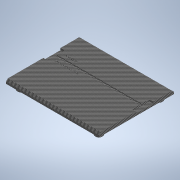
# Autodesk Inventor part: BasePlate2
Saved by Autodesk Inventor 2020 (Build 240168000, 168)
## iProperties
Created: 2026-05-21
Part Number: BasePlate2
Material: Generic
Document SubType Name: Modeling
Designer: sutan
Density: 1 g/cm^3
Appearance: Default
Author: sutan
Autodesk Inventor part; units mm, degrees
ref_plane "YZ Plane" through (0, 0, 0) normal (1, 0, 0) x (0, 1, 0)
ref_plane "XZ Plane" through (0, 0, 0) normal (0, 1, 0) x (-1, 0, 0)
ref_plane "XY Plane" through (0, 0, 0) normal (0, 0, 1) x (1, 0, 0)
sketch "Sketch1" plane through (0, 0, 0) normal (0, 1, 0) x (-1, 0, 0)
  line L0 (22.2515, 145.4131) -> (-225.0785, 145.4131)
  line L1 (-225.0785, 145.4131) -> (-225.0785, 345.4131)
  line L2 (-225.0785, 345.4131) -> (22.2515, 345.4131)
  line L3 (22.2515, 345.4131) -> (22.2515, 145.4131)
  point P0 (0, 0)
  dimension "d0" = 247.33
  dimension "d1" = 200
  constraints: 8 end point, 2 parallel, 1 horizontal, 1 perpendicular
  measures "d0" distance of L1.end L2.end
  measures "d1" distance of L0.end L1.end
extrude "Extrusion1" add sketch "Sketch1" along normal blind 10
sketch "Sketch2" plane through (0, 10, 0) normal (0, 1, 0) x (1, 0, 0)
  line L0 (225.0785, -145.4131) -> (-22.2515, -145.4131) projected
  line L1 (-22.2515, -245.9131) -> (-11.7515, -245.9131)
  line L2 (-11.7515, -245.9131) -> (-11.7515, -200.4131)
  line L3 (-11.7515, -200.4131) -> (-22.2515, -200.4131)
  line L4 (-22.2515, -200.4131) -> (-22.2515, -245.9131)
  line L5 (225.0785, -245.9131) -> (214.5785, -245.9131)
  line L6 (214.5785, -245.9131) -> (214.5785, -200.4131)
  line L7 (214.5785, -200.4131) -> (225.0785, -200.4131)
  line L8 (225.0785, -200.4131) -> (225.0785, -245.9131)
  line L9 (225.0785, -345.4131) -> (225.0785, -145.4131) projected
  line L10 (-22.2515, -145.4131) -> (-22.2515, -345.4131) projected
  point P0 (0, 0)
  point P1 (-9.7325, -245.4131)
  dimension "d4" = 100
  dimension "d5" = 10.5
  dimension "d6" = 45.5
  dimension "d7" = 10.5
  dimension "d8" = 45.5
  dimension "d36" = 0
  dimension "d37" = 0
  dimension "d38" = 0.5
  constraints: 16 end point, 4 parallel, 2 horizontal, 2 perpendicular
  measures "d4" distance from line of L0 point (-9.733, -245.413)
  measures "d5" distance of L3.end L2.end
  measures "d6" distance of L2.end L1.end
  measures "d7" distance of L6.end L7.end
  measures "d8" distance of L5.end L6.end
  measures "d36" distance between parallel lines of L9 L8
  measures "d37" distance between parallel lines of L10 L4
  measures "d38" distance from line of point (-9.733, -245.413) L1
extrude "Extrusion2" cut sketch "Sketch2" against normal blind 5
sketch "Sketch3" plane through (0, 0, 0) normal (0, -1, 0) x (1, 0, 0)
  circle A0 centre (-2.2515, 325.4131) radius 10
  line L0 (-22.2515, 345.4131) -> (225.0785, 345.4131) projected
  line L1 (-22.2515, 145.4131) -> (-22.2515, 345.4131) projected
  line L2 (225.0785, 345.4131) -> (225.0785, 145.4131) projected
  line L3 (225.0785, 145.4131) -> (-22.2515, 145.4131) projected
  circle A1 centre (205.0785, 325.4131) radius 10
  circle A2 centre (205.0785, 165.4131) radius 10
  circle A3 centre (-2.2515, 165.4131) radius 10
  point P0 (0, 0)
  dimension "d11" = 20
  dimension "d12" = 20
  dimension "d13" = 20
  dimension "d16" = 20
  dimension "d17" = 20
  dimension "d18" = 20
  constraints: 4 centre point
  measures "d11" diameter of A0
  measures "d12" distance from line of L0 A0.centre
  measures "d13" distance from line of L1 A0.centre
  measures "d16" diameter of A1
  measures "d17" diameter of A2
  measures "d18" diameter of A3
extrude "Extrusion3" add sketch "Sketch3" along normal blind 15 contours A0 | A1 | A2 | A3
chamfer "Chamfer1" distance 2.5 angle 45 4 edges at (-12.2515, -15, 325.4131) (-12.2515, -15, 165.4131) (195.0785, -15, 325.4131) (195.0785, -15, 165.4131)
sketch "Sketch5" plane through (0, 10, 0) normal (0, 1, 0) x (1, 0, 0)
  line L0 (62.0301, -192.0815) -> (43.5025, -192.0815) construction
  line L1 (43.5025, -192.0815) -> (43.5025, -188.9149) construction
  line L2 (43.5025, -188.9149) -> (62.0301, -188.9149) construction
  line L3 (62.0301, -188.9149) -> (62.0301, -192.0815) construction
  line L4 (-11.7515, -200.4131) -> (-11.7515, -245.9131) projected
  line L5 (214.5785, -245.9131) -> (214.5785, -200.4131) projected
  line L6 (-11.7515, -225.6631) -> (214.5785, -225.6631)
  line L7 (214.5785, -225.6631) -> (214.5785, -220.6631)
  line L8 (214.5785, -220.6631) -> (-11.7515, -220.6631)
  line L9 (-11.7515, -220.6631) -> (-11.7515, -225.6631)
  point P0 (0, 0)
  point P1 (-11.7515, -223.1631)
  point P2 (-11.7515, -220.6631)
  point P3 (214.5785, -225.6631)
  dimension "d24" = 5
  dimension "d25" = 2.5
  constraints: 8 end point, 2 parallel, 2 point on line, 1 horizontal, 1 midpoint, 1 perpendicular, 2 other
  measures "d24" distance of L7.end L6.end
  measures "d25" distance from line of L8 point (-11.751, -223.163)
extrude "Extrusion4" cut sketch "Sketch5" against normal blind 2.5
sketch "Sketch6" plane through (0, 10, 0) normal (0, 1, 0) x (1, 0, 0)
  line L0 (32.5394, -213.5733) -> (0.1071, -213.5733) construction
  line L1 (0.1071, -213.5733) -> (0.1071, -208.0061) construction
  line L2 (0.1071, -208.0061) -> (32.5394, -208.0061) construction
  line L3 (32.5394, -208.0061) -> (32.5394, -213.5733) construction
  line L4 (0.0229, -233.3602) -> (63.709, -233.3602) construction
  line L5 (63.709, -233.3602) -> (63.709, -238.3302) construction
  line L6 (63.709, -238.3302) -> (0.0229, -238.3302) construction
  line L7 (0.0229, -238.3302) -> (0.0229, -233.3602) construction
  spline S0 degree 2 poles (27.8473, -208.5126) (28.1755, -208.3789) (29.2249, -208.1236) (29.7355, -208.1236) knots 0 0 0 1 2 2 2
  spline S1 degree 2 poles (29.7355, -208.1236) (30.9146, -208.1236) (32.3125, -209.485) (32.3125, -210.733) knots 0 0 0 1 2 2 2
  spline S2 degree 2 poles (32.3125, -210.733) (32.3125, -211.9081) (30.9146, -213.3262) (29.699, -213.3262) knots 0 0 0 1 2 2 2
  spline S3 degree 2 poles (29.699, -213.3262) (29.071, -213.3262) (28.2849, -213.0871) (27.8676, -212.8846) knots 0 0 0 1 2 2 2
  line L8 (27.8676, -212.8846) -> (27.8676, -211.7095)
  line L9 (27.8676, -211.7095) -> (27.981, -211.7095)
  spline S4 degree 2 poles (27.981, -211.7095) (28.0702, -211.7784) (28.4105, -212.0418) (28.5726, -212.1309) knots 0 0 0 1 2 2 2
  spline S5 degree 2 poles (28.5726, -212.1309) (28.759, -212.2403) (29.2533, -212.3943) (29.5288, -212.3943) knots 0 0 0 1 2 2 2
  spline S6 degree 2 poles (29.5288, -212.3943) (29.8489, -212.3943) (30.3797, -212.1917) (30.5864, -211.985) knots 0 0 0 1 2 2 2
  spline S7 degree 2 poles (30.5864, -211.985) (30.7849, -211.7824) (31.0159, -211.1625) (31.0159, -210.7533) knots 0 0 0 1 2 2 2
  spline S8 degree 2 poles (31.0159, -210.7533) (31.0159, -209.8781) (30.1366, -209.0434) (29.3789, -209.0434) knots 0 0 0 1 2 2 2
  spline S9 degree 2 poles (29.3789, -209.0434) (29.31, -209.0434) (29.1318, -209.0515) (29.0629, -209.0555) knots 0 0 0 1 2 2 2
  line L10 (29.0629, -209.0555) -> (29.0629, -210.0401)
  line L11 (29.0629, -210.0401) -> (30.0313, -210.0401)
  line L12 (30.0313, -210.0401) -> (30.0313, -210.9761)
  line L13 (30.0313, -210.9761) -> (27.8473, -210.9761)
  line L14 (27.8473, -210.9761) -> (27.8473, -208.5126)
  spline S10 degree 2 poles (23.054, -211.6528) (23.054, -211.3043) (23.2768, -210.6722) (23.4835, -210.4615) knots 0 0 0 1 2 2 2
  spline S11 degree 2 poles (23.4835, -210.4615) (23.6091, -210.3278) (23.917, -210.109) (24.0993, -210.032) knots 0 0 0 1 2 2 2
  spline S12 degree 2 poles (24.0993, -210.032) (24.2857, -209.9551) (24.7193, -209.8659) (24.9867, -209.8659) knots 0 0 0 1 2 2 2
  line L15 (24.9867, -209.8659) -> (25.6431, -209.8659)
  line L16 (25.6431, -209.8659) -> (25.6431, -208.229)
  line L17 (25.6431, -208.229) -> (26.8992, -208.229)
  line L18 (26.8992, -208.229) -> (26.8992, -213.229)
  line L19 (26.8992, -213.229) -> (24.9583, -213.229)
  spline S13 degree 2 poles (24.9583, -213.229) (24.5288, -213.229) (23.9008, -213.0709) (23.6455, -212.9008) knots 0 0 0 1 2 2 2
  spline S14 degree 2 poles (23.6455, -212.9008) (23.3619, -212.7103) (23.054, -212.0863) (23.054, -211.6528) knots 0 0 0 1 2 2 2
  spline S15 degree 2 poles (24.3424, -211.6204) (24.3424, -211.8351) (24.545, -212.139) (24.6828, -212.1957) knots 0 0 0 1 2 2 2
  spline S16 degree 2 poles (24.6828, -212.1957) (24.8611, -212.2727) (25.1852, -212.297) (25.4648, -212.297) knots 0 0 0 1 2 2 2
  line L20 (25.4648, -212.297) -> (25.6431, -212.297)
  line L21 (25.6431, -212.297) -> (25.6431, -210.7978)
  line L22 (25.6431, -210.7978) -> (25.554, -210.7978)
  spline S17 degree 2 poles (25.554, -210.7978) (25.3797, -210.7978) (25.0637, -210.8059) (24.9462, -210.8262) knots 0 0 0 1 2 2 2
  spline S18 degree 2 poles (24.9462, -210.8262) (24.8449, -210.8424) (24.622, -210.9397) (24.5612, -211.0004) knots 0 0 0 1 2 2 2
  spline S19 degree 2 poles (24.5612, -211.0004) (24.4316, -211.122) (24.3424, -211.3935) (24.3424, -211.6204) knots 0 0 0 1 2 2 2
  spline S20 degree 2 poles (20.3595, -208.1236) (21.3684, -208.1236) (22.4543, -209.0961) (22.4543, -210.0361) knots 0 0 0 1 2 2 2
  line L23 (22.4543, -210.0361) -> (22.4543, -213.229)
  line L24 (22.4543, -213.229) -> (21.1982, -213.229)
  line L25 (21.1982, -213.229) -> (21.1982, -210.109)
  spline S21 degree 2 poles (21.1982, -210.109) (21.1982, -209.5863) (20.8052, -209.0758) (20.3595, -209.0758) knots 0 0 0 1 2 2 2
  spline S22 degree 2 poles (20.3595, -209.0758) (19.9259, -209.0758) (19.5207, -209.5661) (19.5207, -210.109) knots 0 0 0 1 2 2 2
  line L26 (19.5207, -210.109) -> (19.5207, -213.229)
  line L27 (19.5207, -213.229) -> (18.2647, -213.229)
  line L28 (18.2647, -213.229) -> (18.2647, -210.0401)
  spline S23 degree 2 poles (18.2647, -210.0401) (18.2647, -209.1163) (19.3222, -208.1236) (20.3595, -208.1236) knots 0 0 0 1 2 2 2
  line L29 (15.2258, -209.9713) -> (17.4502, -209.9713)
  line L30 (17.4502, -209.9713) -> (17.4502, -210.9032)
  line L31 (17.4502, -210.9032) -> (15.2258, -210.9032)
  line L32 (15.2258, -210.9032) -> (15.2258, -209.9713)
  spline S24 degree 2 poles (12.7906, -208.1398) (13.366, -208.1398) (14.233, -208.3627) (14.6058, -208.5247) knots 0 0 0 1 2 2 2
  line L33 (14.6058, -208.5247) -> (14.6058, -209.716)
  line L34 (14.6058, -209.716) -> (14.4924, -209.716)
  spline S25 degree 2 poles (14.4924, -209.716) (14.1155, -209.3959) (13.212, -209.0515) (12.7865, -209.0515) knots 0 0 0 1 2 2 2
  spline S26 degree 2 poles (12.7865, -209.0515) (12.6771, -209.0515) (12.3246, -209.1001) (12.2193, -209.1487) knots 0 0 0 1 2 2 2
  spline S27 degree 2 poles (12.2193, -209.1487) (12.0896, -209.2055) (11.9073, -209.4121) (11.9073, -209.5782) knots 0 0 0 1 2 2 2
  spline S28 degree 2 poles (11.9073, -209.5782) (11.9073, -209.7687) (12.2031, -210.0037) (12.4057, -210.0564) knots 0 0 0 1 2 2 2
  spline S29 degree 2 poles (12.4057, -210.0564) (12.6609, -210.1252) (13.2403, -210.2427) (13.4956, -210.3319) knots 0 0 0 1 2 2 2
  spline S30 degree 2 poles (13.4956, -210.3319) (14.075, -210.5345) (14.5775, -211.2273) (14.5775, -211.746) knots 0 0 0 1 2 2 2
  spline S31 degree 2 poles (14.5775, -211.746) (14.5775, -212.447) (13.3903, -213.3181) (12.4989, -213.3181) knots 0 0 0 1 2 2 2
  spline S32 degree 2 poles (12.4989, -213.3181) (12.0531, -213.3181) (11.1698, -213.1358) (10.8214, -212.9818) knots 0 0 0 1 2 2 2
  line L35 (10.8214, -212.9818) -> (10.8214, -211.8392)
  line L36 (10.8214, -211.8392) -> (10.9308, -211.8392)
  spline S33 degree 2 poles (10.9308, -211.8392) (11.2104, -212.0782) (12.0126, -212.4064) (12.434, -212.4064) knots 0 0 0 1 2 2 2
  spline S34 degree 2 poles (12.434, -212.4064) (12.6001, -212.4064) (12.8595, -212.3578) (13.0053, -212.293) knots 0 0 0 1 2 2 2
  spline S35 degree 2 poles (13.0053, -212.293) (13.1228, -212.2403) (13.293, -212.0296) (13.293, -211.8999) knots 0 0 0 1 2 2 2
  spline S36 degree 2 poles (13.293, -211.8999) (13.293, -211.7055) (13.0215, -211.4826) (12.6326, -211.3935) knots 0 0 0 1 2 2 2
  spline S37 degree 2 poles (12.6326, -211.3935) (12.3813, -211.3367) (11.9154, -211.2273) (11.648, -211.1341) knots 0 0 0 1 2 2 2
  spline S38 degree 2 poles (11.648, -211.1341) (11.1293, -210.9437) (10.6228, -210.3116) (10.6228, -209.793) knots 0 0 0 1 2 2 2
  spline S39 degree 2 poles (10.6228, -209.793) (10.6228, -209.0474) (11.7938, -208.1398) (12.7906, -208.1398) knots 0 0 0 1 2 2 2
  line L37 (8.8724, -208.229) -> (10.0475, -208.229)
  line L38 (10.0475, -208.229) -> (10.0475, -212.0012)
  line L39 (10.0475, -212.0012) -> (8.8724, -212.0012)
  line L40 (8.8724, -212.0012) -> (8.8724, -208.229)
  line L41 (8.836, -212.5401) -> (10.0799, -212.5401)
  line L42 (10.0799, -212.5401) -> (10.0799, -213.4559)
  line L43 (10.0799, -213.4559) -> (8.836, -213.4559)
  line L44 (8.836, -213.4559) -> (8.836, -212.5401)
  line L45 (4.545, -208.229) -> (5.7201, -208.229)
  line L46 (5.7201, -208.229) -> (5.7201, -208.622)
  spline S40 degree 2 poles (5.7201, -208.622) (5.8335, -208.5288) (6.1253, -208.314) (6.2387, -208.2573) knots 0 0 0 1 2 2 2
  spline S41 degree 2 poles (6.2387, -208.2573) (6.3765, -208.1925) (6.652, -208.1236) (6.8424, -208.1236) knots 0 0 0 1 2 2 2
  spline S42 degree 2 poles (6.8424, -208.1236) (7.4867, -208.1236) (8.2403, -209.1933) (8.2403, -210.0847) knots 0 0 0 1 2 2 2
  spline S43 degree 2 poles (8.2403, -210.0847) (8.2403, -210.579) (7.9851, -211.3043) (7.7622, -211.5717) knots 0 0 0 1 2 2 2
  spline S44 degree 2 poles (7.7622, -211.5717) (7.5556, -211.8189) (6.9721, -212.1025) (6.648, -212.1025) knots 0 0 0 1 2 2 2
  spline S45 degree 2 poles (6.648, -212.1025) (6.3522, -212.1025) (5.9713, -211.9769) (5.7201, -211.8473) knots 0 0 0 1 2 2 2
  line L47 (5.7201, -211.8473) -> (5.7201, -213.4518)
  line L48 (5.7201, -213.4518) -> (4.545, -213.4518)
  line L49 (4.545, -213.4518) -> (4.545, -208.229)
  line L50 (5.7201, -209.2662) -> (5.7201, -211.1179)
  spline S46 degree 2 poles (5.7201, -211.1179) (5.8052, -211.1625) (6.0888, -211.2192) (6.1901, -211.2192) knots 0 0 0 1 2 2 2
  spline S47 degree 2 poles (6.1901, -211.2192) (6.6115, -211.2192) (7.0369, -210.6277) (7.0369, -210.0969) knots 0 0 0 1 2 2 2
  spline S48 degree 2 poles (7.0369, -210.0969) (7.0369, -209.5377) (6.6966, -209.0393) (6.3198, -209.0393) knots 0 0 0 1 2 2 2
  spline S49 degree 2 poles (6.3198, -209.0393) (6.1658, -209.0393) (5.8497, -209.1609) (5.7201, -209.2662) knots 0 0 0 1 2 2 2
  spline S50 degree 2 poles (1.7128, -208.1277) (2.7825, -208.1277) (3.9211, -209.1487) (3.9211, -210.0928) knots 0 0 0 1 2 2 2
  spline S51 degree 2 poles (3.9211, -210.0928) (3.9211, -211.0166) (2.8595, -212.1187) (1.9032, -212.1187) knots 0 0 0 1 2 2 2
  spline S52 degree 2 poles (1.9032, -212.1187) (1.0402, -212.1187) (0.165, -211.1828) (0.165, -210.3157) knots 0 0 0 1 2 2 2
  line L51 (0.165, -210.3157) -> (0.165, -209.8902)
  line L52 (0.165, -209.8902) -> (2.746, -209.8902)
  spline S53 degree 2 poles (2.746, -209.8902) (2.7298, -209.6269) (2.5394, -209.2784) (2.3854, -209.173) knots 0 0 0 1 2 2 2
  spline S54 degree 2 poles (2.3854, -209.173) (2.2355, -209.0677) (1.8303, -208.9786) (1.5912, -208.9786) knots 0 0 0 1 2 2 2
  spline S55 degree 2 poles (1.5912, -208.9786) (1.3886, -208.9786) (0.9916, -209.0677) (0.8254, -209.1447) knots 0 0 0 1 2 2 2
  spline S56 degree 2 poles (0.8254, -209.1447) (0.6796, -209.2055) (0.4365, -209.3554) (0.3595, -209.4121) knots 0 0 0 1 2 2 2
  line L53 (0.3595, -209.4121) -> (0.2339, -209.4121)
  line L54 (0.2339, -209.4121) -> (0.2339, -208.4397)
  spline S57 degree 2 poles (0.2339, -208.4397) (0.3797, -208.3829) (0.6147, -208.2857) (0.8254, -208.2371) knots 0 0 0 1 2 2 2
  spline S58 degree 2 poles (0.8254, -208.2371) (1.0159, -208.1844) (1.4211, -208.1277) (1.7128, -208.1277) knots 0 0 0 1 2 2 2
  spline S59 degree 2 poles (1.3238, -210.5993) (1.3319, -210.9721) (1.6601, -211.3651) (1.9964, -211.3651) knots 0 0 0 1 2 2 2
  spline S60 degree 2 poles (1.9964, -211.3651) (2.3408, -211.3651) (2.7298, -210.9518) (2.7501, -210.5993) knots 0 0 0 1 2 2 2
  line L55 (2.7501, -210.5993) -> (1.3238, -210.5993)
  line L56 (5.6469, -238.3999) -> (4.3989, -238.3999)
  line L57 (4.3989, -238.3999) -> (4.3989, -235.0855)
  line L58 (4.3989, -235.0855) -> (3.4913, -237.2249)
  line L59 (3.4913, -237.2249) -> (2.6323, -237.2249)
  line L60 (2.6323, -237.2249) -> (1.7247, -235.0855)
  line L61 (1.7247, -235.0855) -> (1.7247, -238.3999)
  line L62 (1.7247, -238.3999) -> (0.5415, -238.3999)
  line L63 (0.5415, -238.3999) -> (0.5415, -233.3999)
  line L64 (0.5415, -233.3999) -> (1.988, -233.3999)
  line L65 (1.988, -233.3999) -> (3.0982, -235.8675)
  line L66 (3.0982, -235.8675) -> (4.2003, -233.3999)
  line L67 (4.2003, -233.3999) -> (5.6469, -233.3999)
  line L68 (5.6469, -233.3999) -> (5.6469, -238.3999)
  spline S61 degree 2 poles (10.2336, -236.5158) (10.2336, -237.4477) (9.2166, -238.5174) (8.2887, -238.5174) knots 0 0 0 1 2 2 2
  spline S62 degree 2 poles (8.2887, -238.5174) (7.3649, -238.5174) (6.3397, -237.4477) (6.3397, -236.5158) knots 0 0 0 1 2 2 2
  spline S63 degree 2 poles (6.3397, -236.5158) (6.3397, -235.5758) (7.3649, -234.5101) (8.2887, -234.5101) knots 0 0 0 1 2 2 2
  spline S64 degree 2 poles (8.2887, -234.5101) (9.2125, -234.5101) (10.2336, -235.5798) (10.2336, -236.5158) knots 0 0 0 1 2 2 2
  spline S65 degree 2 poles (9.0302, -236.5239) (9.0302, -236.1876) (8.9208, -235.7378) (8.8235, -235.6041) knots 0 0 0 1 2 2 2
  spline S66 degree 2 poles (8.8235, -235.6041) (8.7182, -235.4623) (8.4548, -235.3529) (8.2887, -235.3529) knots 0 0 0 1 2 2 2
  spline S67 degree 2 poles (8.2887, -235.3529) (8.1266, -235.3529) (7.8713, -235.4502) (7.766, -235.5879) knots 0 0 0 1 2 2 2
  spline S68 degree 2 poles (7.766, -235.5879) (7.6647, -235.7176) (7.5431, -236.1754) (7.5431, -236.5239) knots 0 0 0 1 2 2 2
  spline S69 degree 2 poles (7.5431, -236.5239) (7.5431, -236.8683) (7.6566, -237.2938) (7.7498, -237.4234) knots 0 0 0 1 2 2 2
  spline S70 degree 2 poles (7.7498, -237.4234) (7.843, -237.5531) (8.1266, -237.6746) (8.2968, -237.6746) knots 0 0 0 1 2 2 2
  spline S71 degree 2 poles (8.2968, -237.6746) (8.4386, -237.6746) (8.7303, -237.5531) (8.8195, -237.4315) knots 0 0 0 1 2 2 2
  spline S72 degree 2 poles (8.8195, -237.4315) (8.9208, -237.2897) (9.0302, -236.8805) (9.0302, -236.5239) knots 0 0 0 1 2 2 2
  spline S73 degree 2 poles (12.3, -238.4729) (11.5828, -238.4729) (10.9264, -237.8813) (10.9264, -237.2087) knots 0 0 0 1 2 2 2
  line L69 (10.9264, -237.2087) -> (10.9264, -235.4461)
  line L70 (10.9264, -235.4461) -> (10.4767, -235.4461)
  line L71 (10.4767, -235.4461) -> (10.4767, -234.6276)
  line L72 (10.4767, -234.6276) -> (10.9264, -234.6276)
  line L73 (10.9264, -234.6276) -> (10.9264, -233.5498)
  line L74 (10.9264, -233.5498) -> (12.1015, -233.5498)
  line L75 (12.1015, -233.5498) -> (12.1015, -234.6276)
  line L76 (12.1015, -234.6276) -> (13.236, -234.6276)
  line L77 (13.236, -234.6276) -> (13.236, -235.4461)
  line L78 (13.236, -235.4461) -> (12.1015, -235.4461)
  line L79 (12.1015, -235.4461) -> (12.1015, -236.7873)
  spline S74 degree 2 poles (12.1015, -236.7873) (12.1015, -236.9858) (12.1096, -237.2816) (12.1582, -237.3991) knots 0 0 0 1 2 2 2
  spline S75 degree 2 poles (12.1582, -237.3991) (12.2068, -237.5166) (12.4459, -237.6544) (12.6728, -237.6544) knots 0 0 0 1 2 2 2
  spline S76 degree 2 poles (12.6728, -237.6544) (12.77, -237.6544) (13.0739, -237.5733) (13.1347, -237.5409) knots 0 0 0 1 2 2 2
  line L80 (13.1347, -237.5409) -> (13.236, -237.5409)
  line L81 (13.236, -237.5409) -> (13.236, -238.3675)
  spline S77 degree 2 poles (13.236, -238.3675) (13.0456, -238.4161) (12.6161, -238.4729) (12.3, -238.4729) knots 0 0 0 1 2 2 2
  line L82 (17.2433, -238.3999) -> (16.0602, -238.3999)
  line L83 (16.0602, -238.3999) -> (16.0602, -236.532)
  spline S78 degree 2 poles (16.0602, -236.532) (16.0602, -236.3011) (16.0237, -235.8472) (15.9751, -235.7419) knots 0 0 0 1 2 2 2
  spline S79 degree 2 poles (15.9751, -235.7419) (15.9143, -235.6122) (15.6874, -235.5028) (15.4929, -235.5028) knots 0 0 0 1 2 2 2
  spline S80 degree 2 poles (15.4929, -235.5028) (15.3511, -235.5028) (15.0553, -235.6122) (14.8892, -235.7297) knots 0 0 0 1 2 2 2
  line L84 (14.8892, -235.7297) -> (14.8892, -238.3999)
  line L85 (14.8892, -238.3999) -> (13.7141, -238.3999)
  line L86 (13.7141, -238.3999) -> (13.7141, -233.1771)
  line L87 (13.7141, -233.1771) -> (14.8892, -233.1771)
  line L88 (14.8892, -233.1771) -> (14.8892, -235.045)
  spline S81 degree 2 poles (14.8892, -235.045) (15.1768, -234.8019) (15.7238, -234.5263) (16.0561, -234.5263) knots 0 0 0 1 2 2 2
  spline S82 degree 2 poles (16.0561, -234.5263) (16.6315, -234.5263) (17.2433, -235.2557) (17.2433, -235.9445) knots 0 0 0 1 2 2 2
  line L89 (17.2433, -235.9445) -> (17.2433, -238.3999)
  spline S83 degree 2 poles (20.0472, -238.5012) (18.9775, -238.5012) (17.8389, -237.4801) (17.8389, -236.5361) knots 0 0 0 1 2 2 2
  spline S84 degree 2 poles (17.8389, -236.5361) (17.8389, -235.6122) (18.9005, -234.5101) (19.8567, -234.5101) knots 0 0 0 1 2 2 2
  spline S85 degree 2 poles (19.8567, -234.5101) (20.7198, -234.5101) (21.595, -235.4461) (21.595, -236.3132) knots 0 0 0 1 2 2 2
  line L90 (21.595, -236.3132) -> (21.595, -236.7387)
  line L91 (21.595, -236.7387) -> (19.014, -236.7387)
  spline S86 degree 2 poles (19.014, -236.7387) (19.0302, -237.002) (19.2206, -237.3505) (19.3746, -237.4558) knots 0 0 0 1 2 2 2
  spline S87 degree 2 poles (19.3746, -237.4558) (19.5245, -237.5612) (19.9297, -237.6503) (20.1687, -237.6503) knots 0 0 0 1 2 2 2
  spline S88 degree 2 poles (20.1687, -237.6503) (20.3713, -237.6503) (20.7684, -237.5612) (20.9345, -237.4842) knots 0 0 0 1 2 2 2
  spline S89 degree 2 poles (20.9345, -237.4842) (21.0804, -237.4234) (21.3235, -237.2735) (21.4005, -237.2168) knots 0 0 0 1 2 2 2
  line L92 (21.4005, -237.2168) -> (21.5261, -237.2168)
  line L93 (21.5261, -237.2168) -> (21.5261, -238.1892)
  spline S90 degree 2 poles (21.5261, -238.1892) (21.3803, -238.246) (21.1452, -238.3432) (20.9345, -238.3918) knots 0 0 0 1 2 2 2
  spline S91 degree 2 poles (20.9345, -238.3918) (20.7441, -238.4445) (20.3389, -238.5012) (20.0472, -238.5012) knots 0 0 0 1 2 2 2
  spline S92 degree 2 poles (20.4362, -236.0296) (20.4281, -235.6568) (20.0999, -235.2638) (19.7636, -235.2638) knots 0 0 0 1 2 2 2
  spline S93 degree 2 poles (19.7636, -235.2638) (19.4191, -235.2638) (19.0302, -235.6771) (19.0099, -236.0296) knots 0 0 0 1 2 2 2
  line L94 (19.0099, -236.0296) -> (20.4362, -236.0296)
  line L95 (24.7311, -235.7419) -> (24.6339, -235.7419)
  spline S94 degree 2 poles (24.6339, -235.7419) (24.565, -235.7176) (24.3097, -235.6933) (24.1558, -235.6933) knots 0 0 0 1 2 2 2
  spline S95 degree 2 poles (24.1558, -235.6933) (23.9734, -235.6933) (23.5642, -235.8027) (23.3738, -235.8756) knots 0 0 0 1 2 2 2
  line L96 (23.3738, -235.8756) -> (23.3738, -238.3999)
  line L97 (23.3738, -238.3999) -> (22.1987, -238.3999)
  line L98 (22.1987, -238.3999) -> (22.1987, -234.6276)
  line L99 (22.1987, -234.6276) -> (23.3738, -234.6276)
  line L100 (23.3738, -234.6276) -> (23.3738, -235.1706)
  spline S96 degree 2 poles (23.3738, -235.1706) (23.4548, -235.0977) (23.7384, -234.8707) (23.8559, -234.8019) knots 0 0 0 1 2 2 2
  spline S97 degree 2 poles (23.8559, -234.8019) (23.9856, -234.7249) (24.326, -234.6155) (24.4759, -234.6155) knots 0 0 0 1 2 2 2
  spline S98 degree 2 poles (24.4759, -234.6155) (24.5326, -234.6155) (24.6744, -234.6236) (24.7311, -234.6276) knots 0 0 0 1 2 2 2
  line L101 (24.7311, -234.6276) -> (24.7311, -235.7419)
  spline S99 degree 2 poles (28.8762, -236.4631) (28.8762, -237.3626) (27.9645, -238.4729) (27.2879, -238.4729) knots 0 0 0 1 2 2 2
  spline S100 degree 2 poles (27.2879, -238.4729) (27.0083, -238.4729) (26.5909, -238.3472) (26.3559, -238.2135) knots 0 0 0 1 2 2 2
  line L102 (26.3559, -238.2135) -> (26.3073, -238.3999)
  line L103 (26.3073, -238.3999) -> (25.1809, -238.3999)
  line L104 (25.1809, -238.3999) -> (25.1809, -233.1771)
  line L105 (25.1809, -233.1771) -> (26.3559, -233.1771)
  line L106 (26.3559, -233.1771) -> (26.3559, -235.0247)
  spline S101 degree 2 poles (26.3559, -235.0247) (26.6153, -234.8019) (27.1501, -234.5263) (27.5026, -234.5263) knots 0 0 0 1 2 2 2
  spline S102 degree 2 poles (27.5026, -234.5263) (28.1631, -234.5263) (28.8762, -235.5515) (28.8762, -236.4631) knots 0 0 0 1 2 2 2
  spline S103 degree 2 poles (27.6728, -236.4874) (27.6728, -235.9242) (27.3324, -235.4421) (26.9759, -235.4421) knots 0 0 0 1 2 2 2
  spline S104 degree 2 poles (26.9759, -235.4421) (26.8179, -235.4421) (26.5059, -235.5434) (26.3559, -235.6447) knots 0 0 0 1 2 2 2
  line L107 (26.3559, -235.6447) -> (26.3559, -237.5328)
  spline S105 degree 2 poles (26.3559, -237.5328) (26.4734, -237.5814) (26.7125, -237.6139) (26.83, -237.6139) knots 0 0 0 1 2 2 2
  spline S106 degree 2 poles (26.83, -237.6139) (27.2555, -237.6139) (27.6728, -237.0507) (27.6728, -236.4874) knots 0 0 0 1 2 2 2
  spline S107 degree 2 poles (33.1428, -236.5158) (33.1428, -237.4477) (32.1258, -238.5174) (31.1979, -238.5174) knots 0 0 0 1 2 2 2
  spline S108 degree 2 poles (31.1979, -238.5174) (30.2741, -238.5174) (29.249, -237.4477) (29.249, -236.5158) knots 0 0 0 1 2 2 2
  spline S109 degree 2 poles (29.249, -236.5158) (29.249, -235.5758) (30.2741, -234.5101) (31.1979, -234.5101) knots 0 0 0 1 2 2 2
  spline S110 degree 2 poles (31.1979, -234.5101) (32.1217, -234.5101) (33.1428, -235.5798) (33.1428, -236.5158) knots 0 0 0 1 2 2 2
  spline S111 degree 2 poles (31.9394, -236.5239) (31.9394, -236.1876) (31.83, -235.7378) (31.7328, -235.6041) knots 0 0 0 1 2 2 2
  spline S112 degree 2 poles (31.7328, -235.6041) (31.6274, -235.4623) (31.364, -235.3529) (31.1979, -235.3529) knots 0 0 0 1 2 2 2
  spline S113 degree 2 poles (31.1979, -235.3529) (31.0358, -235.3529) (30.7806, -235.4502) (30.6752, -235.5879) knots 0 0 0 1 2 2 2
  spline S114 degree 2 poles (30.6752, -235.5879) (30.5739, -235.7176) (30.4524, -236.1754) (30.4524, -236.5239) knots 0 0 0 1 2 2 2
  spline S115 degree 2 poles (30.4524, -236.5239) (30.4524, -236.8683) (30.5658, -237.2938) (30.659, -237.4234) knots 0 0 0 1 2 2 2
  spline S116 degree 2 poles (30.659, -237.4234) (30.7522, -237.5531) (31.0358, -237.6746) (31.206, -237.6746) knots 0 0 0 1 2 2 2
  spline S117 degree 2 poles (31.206, -237.6746) (31.3478, -237.6746) (31.6396, -237.5531) (31.7287, -237.4315) knots 0 0 0 1 2 2 2
  spline S118 degree 2 poles (31.7287, -237.4315) (31.83, -237.2897) (31.9394, -236.8805) (31.9394, -236.5239) knots 0 0 0 1 2 2 2
  spline S119 degree 2 poles (35.8454, -237.9988) (35.7238, -238.1001) (35.5334, -238.2622) (35.3713, -238.3432) knots 0 0 0 1 2 2 2
  spline S120 degree 2 poles (35.3713, -238.3432) (35.2133, -238.4202) (34.9135, -238.5012) (34.6461, -238.5012) knots 0 0 0 1 2 2 2
  spline S121 degree 2 poles (34.6461, -238.5012) (34.1436, -238.5012) (33.4832, -237.8286) (33.4832, -237.3181) knots 0 0 0 1 2 2 2
  spline S122 degree 2 poles (33.4832, -237.3181) (33.4832, -236.9007) (33.8195, -236.3821) (34.1355, -236.2322) knots 0 0 0 1 2 2 2
  spline S123 degree 2 poles (34.1355, -236.2322) (34.4556, -236.0782) (35.343, -235.9566) (35.8535, -235.9242) knots 0 0 0 1 2 2 2
  line L108 (35.8535, -235.9242) -> (35.8535, -235.904)
  spline S124 degree 2 poles (35.8535, -235.904) (35.8535, -235.592) (35.3916, -235.3529) (34.9297, -235.3529) knots 0 0 0 1 2 2 2
  spline S125 degree 2 poles (34.9297, -235.3529) (34.723, -235.3529) (34.1639, -235.5028) (33.9005, -235.6203) knots 0 0 0 1 2 2 2
  line L109 (33.9005, -235.6203) -> (33.7992, -235.6203)
  line L110 (33.7992, -235.6203) -> (33.7992, -234.7087)
  spline S126 degree 2 poles (33.7992, -234.7087) (33.9734, -234.6601) (34.7514, -234.5223) (35.1485, -234.5223) knots 0 0 0 1 2 2 2
  spline S127 degree 2 poles (35.1485, -234.5223) (36.1209, -234.5223) (37.0123, -235.1706) (37.0123, -235.8351) knots 0 0 0 1 2 2 2
  line L111 (37.0123, -235.8351) -> (37.0123, -238.3999)
  line L112 (37.0123, -238.3999) -> (35.8454, -238.3999)
  line L113 (35.8454, -238.3999) -> (35.8454, -237.9988)
  line L114 (35.8454, -237.4153) -> (35.8454, -236.6333)
  spline S128 degree 2 poles (35.8454, -236.6333) (35.5456, -236.6617) (35.1768, -236.7062) (34.9986, -236.7711) knots 0 0 0 1 2 2 2
  spline S129 degree 2 poles (34.9986, -236.7711) (34.8405, -236.8237) (34.6704, -237.0425) (34.6704, -237.2208) knots 0 0 0 1 2 2 2
  spline S130 degree 2 poles (34.6704, -237.2208) (34.6704, -237.4842) (34.958, -237.6827) (35.2376, -237.6827) knots 0 0 0 1 2 2 2
  spline S131 degree 2 poles (35.2376, -237.6827) (35.3916, -237.6827) (35.7157, -237.5409) (35.8454, -237.4153) knots 0 0 0 1 2 2 2
  line L115 (40.4159, -235.7419) -> (40.3187, -235.7419)
  spline S132 degree 2 poles (40.3187, -235.7419) (40.2498, -235.7176) (39.9945, -235.6933) (39.8405, -235.6933) knots 0 0 0 1 2 2 2
  spline S133 degree 2 poles (39.8405, -235.6933) (39.6582, -235.6933) (39.249, -235.8027) (39.0585, -235.8756) knots 0 0 0 1 2 2 2
  line L116 (39.0585, -235.8756) -> (39.0585, -238.3999)
  line L117 (39.0585, -238.3999) -> (37.8835, -238.3999)
  line L118 (37.8835, -238.3999) -> (37.8835, -234.6276)
  line L119 (37.8835, -234.6276) -> (39.0585, -234.6276)
  line L120 (39.0585, -234.6276) -> (39.0585, -235.1706)
  spline S134 degree 2 poles (39.0585, -235.1706) (39.1396, -235.0977) (39.4232, -234.8707) (39.5407, -234.8019) knots 0 0 0 1 2 2 2
  spline S135 degree 2 poles (39.5407, -234.8019) (39.6704, -234.7249) (40.0107, -234.6155) (40.1606, -234.6155) knots 0 0 0 1 2 2 2
  spline S136 degree 2 poles (40.1606, -234.6155) (40.2174, -234.6155) (40.3592, -234.6236) (40.4159, -234.6276) knots 0 0 0 1 2 2 2
  line L121 (40.4159, -234.6276) -> (40.4159, -235.7419)
  line L122 (44.2935, -238.3999) -> (43.1185, -238.3999)
  line L123 (43.1185, -238.3999) -> (43.1185, -238.0069)
  spline S137 degree 2 poles (43.1185, -238.0069) (43.005, -238.1001) (42.7133, -238.3148) (42.5999, -238.3716) knots 0 0 0 1 2 2 2
  spline S138 degree 2 poles (42.5999, -238.3716) (42.4621, -238.4364) (42.1866, -238.5053) (41.9961, -238.5053) knots 0 0 0 1 2 2 2
  spline S139 degree 2 poles (41.9961, -238.5053) (41.3519, -238.5053) (40.5982, -237.4356) (40.5982, -236.5442) knots 0 0 0 1 2 2 2
  spline S140 degree 2 poles (40.5982, -236.5442) (40.5982, -236.0498) (40.8535, -235.3246) (41.0764, -235.0571) knots 0 0 0 1 2 2 2
  spline S141 degree 2 poles (41.0764, -235.0571) (41.283, -234.81) (41.8665, -234.5263) (42.1906, -234.5263) knots 0 0 0 1 2 2 2
  spline S142 degree 2 poles (42.1906, -234.5263) (42.4864, -234.5263) (42.8673, -234.6519) (43.1185, -234.7816) knots 0 0 0 1 2 2 2
  line L124 (43.1185, -234.7816) -> (43.1185, -233.1771)
  line L125 (43.1185, -233.1771) -> (44.2935, -233.1771)
  line L126 (44.2935, -233.1771) -> (44.2935, -238.3999)
  line L127 (43.1185, -237.3626) -> (43.1185, -235.5109)
  spline S143 degree 2 poles (43.1185, -235.5109) (43.0334, -235.4664) (42.7498, -235.4096) (42.6485, -235.4096) knots 0 0 0 1 2 2 2
  spline S144 degree 2 poles (42.6485, -235.4096) (42.2271, -235.4096) (41.8016, -236.0012) (41.8016, -236.532) knots 0 0 0 1 2 2 2
  spline S145 degree 2 poles (41.8016, -236.532) (41.8016, -237.0912) (42.142, -237.5896) (42.5188, -237.5896) knots 0 0 0 1 2 2 2
  spline S146 degree 2 poles (42.5188, -237.5896) (42.6728, -237.5896) (42.9888, -237.468) (43.1185, -237.3626) knots 0 0 0 1 2 2 2
  spline S147 degree 2 poles (48.8195, -238.4891) (48.2441, -238.4891) (47.377, -238.2662) (47.0042, -238.1041) knots 0 0 0 1 2 2 2
  line L128 (47.0042, -238.1041) -> (47.0042, -236.9129)
  line L129 (47.0042, -236.9129) -> (47.1177, -236.9129)
  spline S148 degree 2 poles (47.1177, -236.9129) (47.4945, -237.233) (48.3981, -237.5774) (48.8235, -237.5774) knots 0 0 0 1 2 2 2
  spline S149 degree 2 poles (48.8235, -237.5774) (48.9329, -237.5774) (49.2854, -237.5288) (49.3908, -237.4801) knots 0 0 0 1 2 2 2
  spline S150 degree 2 poles (49.3908, -237.4801) (49.5204, -237.4234) (49.7028, -237.2168) (49.7028, -237.0507) knots 0 0 0 1 2 2 2
  spline S151 degree 2 poles (49.7028, -237.0507) (49.7028, -236.8602) (49.407, -236.6252) (49.2044, -236.5725) knots 0 0 0 1 2 2 2
  spline S152 degree 2 poles (49.2044, -236.5725) (48.9491, -236.5037) (48.3697, -236.3861) (48.1144, -236.297) knots 0 0 0 1 2 2 2
  spline S153 degree 2 poles (48.1144, -236.297) (47.535, -236.0944) (47.0326, -235.4015) (47.0326, -234.8829) knots 0 0 0 1 2 2 2
  spline S154 degree 2 poles (47.0326, -234.8829) (47.0326, -234.1819) (48.2198, -233.3108) (49.1112, -233.3108) knots 0 0 0 1 2 2 2
  spline S155 degree 2 poles (49.1112, -233.3108) (49.5569, -233.3108) (50.4402, -233.4931) (50.7887, -233.6471) knots 0 0 0 1 2 2 2
  line L130 (50.7887, -233.6471) -> (50.7887, -234.7897)
  line L131 (50.7887, -234.7897) -> (50.6793, -234.7897)
  spline S156 degree 2 poles (50.6793, -234.7897) (50.3997, -234.5507) (49.5974, -234.2225) (49.176, -234.2225) knots 0 0 0 1 2 2 2
  spline S157 degree 2 poles (49.176, -234.2225) (49.0099, -234.2225) (48.7506, -234.2711) (48.6047, -234.3359) knots 0 0 0 1 2 2 2
  spline S158 degree 2 poles (48.6047, -234.3359) (48.4872, -234.3886) (48.317, -234.5993) (48.317, -234.7289) knots 0 0 0 1 2 2 2
  spline S159 degree 2 poles (48.317, -234.7289) (48.317, -234.9234) (48.5885, -235.1463) (48.9775, -235.2354) knots 0 0 0 1 2 2 2
  spline S160 degree 2 poles (48.9775, -235.2354) (49.2287, -235.2921) (49.6947, -235.4015) (49.9621, -235.4947) knots 0 0 0 1 2 2 2
  spline S161 degree 2 poles (49.9621, -235.4947) (50.4807, -235.6852) (50.9872, -236.3173) (50.9872, -236.8359) knots 0 0 0 1 2 2 2
  spline S162 degree 2 poles (50.9872, -236.8359) (50.9872, -237.5814) (49.8162, -238.4891) (48.8195, -238.4891) knots 0 0 0 1 2 2 2
  line L132 (52.7376, -238.3999) -> (51.5626, -238.3999)
  line L133 (51.5626, -238.3999) -> (51.5626, -234.6276)
  line L134 (51.5626, -234.6276) -> (52.7376, -234.6276)
  line L135 (52.7376, -234.6276) -> (52.7376, -238.3999)
  line L136 (52.7741, -234.0887) -> (51.5302, -234.0887)
  line L137 (51.5302, -234.0887) -> (51.5302, -233.173)
  line L138 (51.5302, -233.173) -> (52.7741, -233.173)
  line L139 (52.7741, -233.173) -> (52.7741, -234.0887)
  line L140 (57.065, -238.3999) -> (55.89, -238.3999)
  line L141 (55.89, -238.3999) -> (55.89, -238.0069)
  spline S163 degree 2 poles (55.89, -238.0069) (55.7765, -238.1001) (55.4848, -238.3148) (55.3713, -238.3716) knots 0 0 0 1 2 2 2
  spline S164 degree 2 poles (55.3713, -238.3716) (55.2336, -238.4364) (54.958, -238.5053) (54.7676, -238.5053) knots 0 0 0 1 2 2 2
  spline S165 degree 2 poles (54.7676, -238.5053) (54.1234, -238.5053) (53.3697, -237.4356) (53.3697, -236.5442) knots 0 0 0 1 2 2 2
  spline S166 degree 2 poles (53.3697, -236.5442) (53.3697, -236.0498) (53.625, -235.3246) (53.8478, -235.0571) knots 0 0 0 1 2 2 2
  spline S167 degree 2 poles (53.8478, -235.0571) (54.0545, -234.81) (54.6379, -234.5263) (54.9621, -234.5263) knots 0 0 0 1 2 2 2
  spline S168 degree 2 poles (54.9621, -234.5263) (55.2579, -234.5263) (55.6388, -234.6519) (55.89, -234.7816) knots 0 0 0 1 2 2 2
  line L142 (55.89, -234.7816) -> (55.89, -233.1771)
  line L143 (55.89, -233.1771) -> (57.065, -233.1771)
  line L144 (57.065, -233.1771) -> (57.065, -238.3999)
  line L145 (55.89, -237.3626) -> (55.89, -235.5109)
  spline S169 degree 2 poles (55.89, -235.5109) (55.8049, -235.4664) (55.5213, -235.4096) (55.42, -235.4096) knots 0 0 0 1 2 2 2
  spline S170 degree 2 poles (55.42, -235.4096) (54.9986, -235.4096) (54.5731, -236.0012) (54.5731, -236.532) knots 0 0 0 1 2 2 2
  spline S171 degree 2 poles (54.5731, -236.532) (54.5731, -237.0912) (54.9135, -237.5896) (55.2903, -237.5896) knots 0 0 0 1 2 2 2
  spline S172 degree 2 poles (55.2903, -237.5896) (55.4443, -237.5896) (55.7603, -237.468) (55.89, -237.3626) knots 0 0 0 1 2 2 2
  spline S173 degree 2 poles (59.8973, -238.5012) (58.8276, -238.5012) (57.689, -237.4801) (57.689, -236.5361) knots 0 0 0 1 2 2 2
  spline S174 degree 2 poles (57.689, -236.5361) (57.689, -235.6122) (58.7506, -234.5101) (59.7068, -234.5101) knots 0 0 0 1 2 2 2
  spline S175 degree 2 poles (59.7068, -234.5101) (60.5699, -234.5101) (61.4451, -235.4461) (61.4451, -236.3132) knots 0 0 0 1 2 2 2
  line L146 (61.4451, -236.3132) -> (61.4451, -236.7387)
  line L147 (61.4451, -236.7387) -> (58.864, -236.7387)
  spline S176 degree 2 poles (58.864, -236.7387) (58.8803, -237.002) (59.0707, -237.3505) (59.2247, -237.4558) knots 0 0 0 1 2 2 2
  spline S177 degree 2 poles (59.2247, -237.4558) (59.3746, -237.5612) (59.7798, -237.6503) (60.0188, -237.6503) knots 0 0 0 1 2 2 2
  spline S178 degree 2 poles (60.0188, -237.6503) (60.2214, -237.6503) (60.6185, -237.5612) (60.7846, -237.4842) knots 0 0 0 1 2 2 2
  spline S179 degree 2 poles (60.7846, -237.4842) (60.9305, -237.4234) (61.1736, -237.2735) (61.2506, -237.2168) knots 0 0 0 1 2 2 2
  line L148 (61.2506, -237.2168) -> (61.3762, -237.2168)
  line L149 (61.3762, -237.2168) -> (61.3762, -238.1892)
  spline S180 degree 2 poles (61.3762, -238.1892) (61.2303, -238.246) (60.9953, -238.3432) (60.7846, -238.3918) knots 0 0 0 1 2 2 2
  spline S181 degree 2 poles (60.7846, -238.3918) (60.5942, -238.4445) (60.189, -238.5012) (59.8973, -238.5012) knots 0 0 0 1 2 2 2
  spline S182 degree 2 poles (60.2862, -236.0296) (60.2781, -235.6568) (59.9499, -235.2638) (59.6136, -235.2638) knots 0 0 0 1 2 2 2
  spline S183 degree 2 poles (59.6136, -235.2638) (59.2692, -235.2638) (58.8803, -235.6771) (58.86, -236.0296) knots 0 0 0 1 2 2 2
  line L150 (58.86, -236.0296) -> (60.2862, -236.0296)
  point P0 (0, 0)
  constraints: 4 other
extrude "Extrusion5" cut sketch "Sketch6" against normal blind 2.5
chamfer "Chamfer3" distance 5 angle 45 2 edges at (101.4135, 10, 145.4131) (101.4135, 10, 345.4131)
sketch "Sketch9" plane through (0, 10, 0) normal (0, 1, 0) x (1, 0, 0)
  line L0 (225.0785, -340.4131) -> (-22.2515, -340.4131) projected
  line L1 (51.4135, -340.4131) -> (151.4135, -340.4131)
  line L2 (151.4135, -340.4131) -> (151.4135, -320.4131)
  line L3 (151.4135, -320.4131) -> (51.4135, -320.4131)
  line L4 (51.4135, -320.4131) -> (51.4135, -340.4131)
  line L5 (-22.2515, -245.9131) -> (-22.2515, -340.4131) projected
  point P0 (0, 0)
  point P1 (101.4135, -330.4131)
  dimension "d46" = 100
  dimension "d47" = 20
  dimension "d48" = 123.665
  dimension "d49" = 50
  constraints: 8 end point, 2 parallel, 1 horizontal, 1 perpendicular, 1 point on line
  measures "d46" distance of L3.end L2.end
  measures "d47" distance of L2.end L1.end
  measures "d48" distance from line of L5 point (101.414, -330.413)
  measures "d49" distance from line of L2 point (101.414, -330.413)
extrude "Extrusion7" cut sketch "Sketch9" against normal up to surface (10 mm away)
fillet "Fillet1" radius 2.5 2 edges at (101.4135, 10, 340.4131) (101.4135, 0, 340.4131)
chamfer "Chamfer4" distance 2.5 angle 45 2 edges at (51.4135, 5, 320.4131) (151.4135, 5, 320.4131)
equation "\"d4\" = 0.5 * d1"
equation "\"d7\" = d5"
equation "\"d8\" = d6"
equation "\"d25\" = 0.5 * d24"
equation "\"d26\" = 0.5 * d9"
equation "\"d31\" = 0.5 * d9"
equation "\"d48\" = 0.5 * d0"
equation "\"d49\" = 0.5 * d46"
equation "\"d9\" = 5"
body "Solid1"
